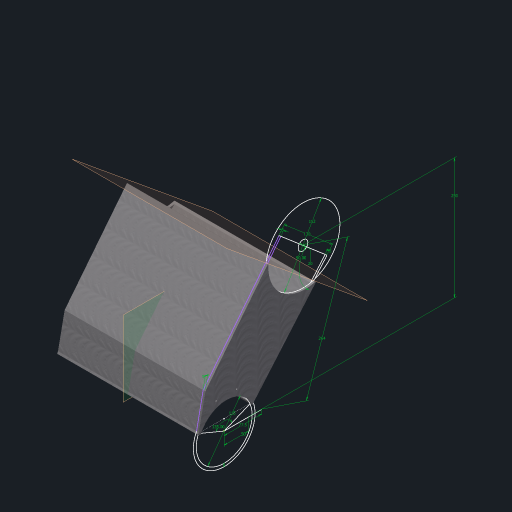
# Autodesk Inventor part: CANALETA_GUIA
Saved by Autodesk Inventor 2024.3 (Build 283343000, 343)
## iProperties
Created: 2024-07-12
Part Number: CANALETA_GUIA
Material: Steel, Mild, Welded
Document SubType Name: Modeling
Designer: Niler
Density: 7.85 g/cm^3
Appearance: Weld - Steel Mild
Author: Niler
Autodesk Inventor part; units mm, degrees
ref_plane "YZ Plane" through (0, 0, 0) normal (1, 0, 0) x (0, 1, 0)
ref_plane "XZ Plane" through (0, 0, 0) normal (0, 1, 0) x (-1, 0, 0)
ref_plane "XY Plane" through (0, 0, 0) normal (0, 0, 1) x (1, 0, 0)
sketch "Sketch1" plane through (0, 0, 0) normal (1, 0, 0) x (0, 1, 0)
  circle A0 centre (0, 0) radius 57.5
  line L0 (0, 0) -> (22.0043, 53.1231)
  line L1 (0, 0) -> (22.0043, -53.1231)
  line L2 (22.0043, 53.1231) -> (22.0043, -53.1231) construction
  line L3 (22.0043, 53.1231) -> (24.3004, 58.6664)
  line L4 (22.0043, -53.1231) -> (24.3004, -58.6664)
  circle A1 centre (0, 0) radius 63.5
  line L5 (22.0043, -53.1231) -> (207.792, -211.7609)
  line L6 (0, 0) -> (0, -50)
  line L7 (94.6424, 43.3552) -> (292.208, -112.8976)
  line L8 (92.474, 38.6955) -> (288.9589, -116.7027)
  line L9 (26.9658, -50.7848) -> (211.0388, -207.9584)
  line L10 (292.208, -112.8976) -> (207.792, -211.7609)
  circle A2 centre (250, -162.3292) radius 10
  circle A3 centre (250, -162.3292) radius 76
  line L11 (94.6424, 43.3552) -> (27.9796, 57.0034)
  line L12 (22.0043, 53.1231) -> (92.474, 38.6955)
  line L13 (0, 0) -> (0, -77.5)
  point P0 (22.0043, 0)
  point P1 (250.5574, -86.3313)
  point P2 (259.3441, -86.9058)
  point P3 (177.842, -186.1875)
  point P4 (175.5639, -177.6676)
  point P5 (243.5065, -169.9341)
  point P6 (256.4935, -154.7244)
  point P7 (27.0643, -57.4436)
  point P8 (39.7995, 49.4798)
  point P9 (31.8357, -54.943)
  dimension "d0" = 115
  dimension "d1" = 135
  dimension "d2" = 6
  dimension "d6" = 5
  dimension "d7" = 5
  dimension "d8" = 90
  dimension "d9" = 130
  dimension "d11" = 50
  dimension "d14" = 20
  dimension "d16" = 152
  dimension "d17" = 250
  dimension "d18" = 5
  dimension "d24" = 77.5
  dimension "d26" = 264
  constraints: 28 end point, 6 point on circle, 4 centre point, 3 coincident, 3 parallel, 3 point on line, 2 midpoint, 2 vertical, 1 collinear, 1 horizontal alignment
  measures "d0" diameter of A0
  measures "d1" angle of L0 L1
  measures "d2" radial gap between concentric circles of A0 A1
  measures "d6" distance between parallel lines of L8 L7
  measures "d7" distance between parallel lines of L5 L9
  measures "d8" angle of L10 L5
  measures "d9" distance of L7.end L5.end
  measures "d11" distance of L0.start L6.end
  measures "d14" diameter of A2
  measures "d16" diameter of A3
  measures "d17" distance from line of A2.centre L6
  measures "d18" distance between parallel lines of L11 L12
  measures "d24" distance of L0.start L13.end
  measures "d26" distance of A2.centre L13.end
extrude "Extrusion1" add sketch "Sketch1" against normal blind 280 contours L3 A1 L12 | L9 A1 L5 A0 | A1 L11 L7 A3 L8 L12 | L9 A3 L5 A1
extrude "Extrusion2" add sketch "Sketch1" along normal blind 5 contours A0 L12 A1 L9 | L3 A1 L12 | L9 A1 L5 A0 | L12 L8 A3 L9 A1 | A1 L11 L7 A3 L8 L12 | L9 A3 L5 A1
ref_plane "Work Plane1" through (-140, 0, 0) normal (-1, 0, 0) x (0, 0, 1)
mirror "Mirror1" about plane through (-140, 0, 0) normal (-1, 0, 0) of "Extrusion2"
sketch "Sketch2" plane through (5, 0, 0) normal (1, 0, 0) x (0, 0, -1)
  line L0 (86.9058, 259.3441) -> (-43.3552, 94.6424) projected
  line L1 (-43.3552, 94.6424) -> (-57.0034, 27.9796) projected
  arc A0 (-57.0034, 27.9796) -> (-58.6664, 24.3004) centre (0, 0) ccw projected
  line L2 (-58.6664, 24.3004) -> (-53.1231, 22.0043) projected
  arc A1 (53.1231, 22.0043) -> (-53.1231, 22.0043) centre (0, 0) ccw projected
  line L3 (53.1231, 22.0043) -> (186.1875, 177.842) projected
  arc A2 (86.9058, 259.3441) -> (186.1875, 177.842) centre (162.3292, 250) ccw projected
  circle A3 centre (0, 0) radius 63.5 projected
  circle A4 centre (-21.0494, 66.7602) radius 1.65
  line L4 (-21.0494, 66.7602) -> (0, 0) construction
  line L5 (0, 0) -> (21.0494, 66.7602) construction
  line L6 (-21.0494, 66.7602) -> (21.0494, 66.7602) construction
  circle A5 centre (21.0494, 66.7602) radius 1.65
  point P0 (0, 66.7602)
  dimension "d19" = 3.3
  dimension "d20" = 70
  dimension "d21" = 35
  constraints: 6 end point, 2 centre point, 1 coincident, 1 equal radius, 1 horizontal alignment, 1 midpoint, 1 vertical alignment
  measures "d19" diameter of A4
  measures "d20" distance of L4.start L4.end
  measures "d21" angle of L5 L4
extrude "Extrusion3" cut sketch "Sketch2" against normal through all contours A4 | A5
ref_plane "Work Plane2" through (0, 259.3441, -86.9058) normal (0, 0.7729, -0.6345) x (1, 0, 0)
sketch "Sketch3" plane through (0, 259.3441, -86.9058) normal (0, 0.7729, -0.6345) x (1, 0, 0)
  line L0 (-314.1788, 142.1673) -> (47.7858, 142.1673)
  line L1 (47.7858, 142.1673) -> (47.7858, -28.3874)
  line L2 (47.7858, -28.3874) -> (-314.1788, -28.3874)
  line L3 (-314.1788, -28.3874) -> (-314.1788, 142.1673)
  point P0 (0, 97.3835)
  constraints: 8 end point, 2 parallel, 1 horizontal, 1 perpendicular
extrude "Extrusion4" cut sketch "Sketch3" against normal blind 3
body "Solid1"
